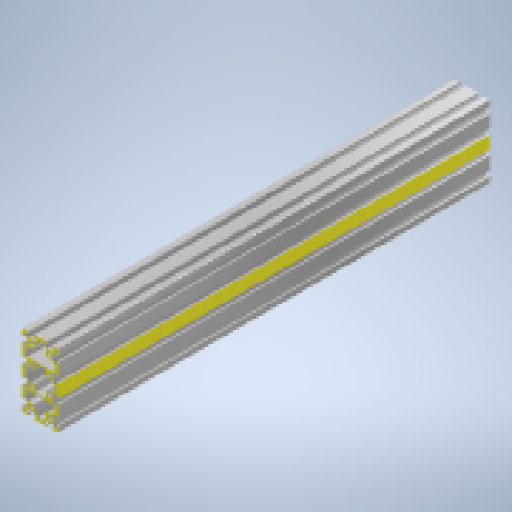
# Autodesk Inventor part: HFS5-4080-495
Saved by Autodesk Inventor 2024 (Build 280153000, 153)
## iProperties
Category: PARTsolutions
Company: MISUMI
Created: 2024-12-16
Part Number: HFS5-4080-495
Material: Aluminum 6061
Catalog Web Link: www.cadenas.de
Description: HFS5-2060, HFS5-2080, HFS5-4060, HFS5-4080, NFS5-2060, NFS5-2080, NFS5-4060, NFS5-4080-HFS5 Series Aluminum Extrusions 20mm Square -3 or more slots-
Vendor: MISUMI
Document SubType Name: Modeling
Designer: psAdmin
Manufacturer: MISUMI
Mass: 1327.09 g
Surface Area: 4398.43 cm^2
Volume: 491.514 cm^3
Density: 2.7 g/cm^3
Appearance: Aluminum - Flat
PSOL_IDENT_0: {$CADENAS_DATA/23d-libs/misumi/metric/38_al_extrusions_blackets/5/hfs5_2060.prj},622 {VTYP=3D},{NB=H
PSOL_IDENT_1: FS5-4080-495},{LINA=HFS5-4080-495},{NN=HFS5-2060, HFS5-2080, HFS5-4060, HFS5-4080, NFS5-2060, NFS5-2
PSOL_IDENT_2: 080, NFS5-4060, NFS5-4080},{DATE=08.05.2023 08:44:46},{GEOMDATE=27.07.2021 03:20:00},{VERSION=},{LIN
PSOL_IDENT_3: EID=220},{WBVAR=L,ALT1,ALT2,ALT4,ALT5,CP5,DL5,DR5,ALT6,ALT9,ALT10,ALT11,HP6,NHL6,DL6,NHR6,DR6,ALT7,A
PSOL_IDENT_4: LT8,NH9,AH,BH,CH,DH,EH,NH10,AV,BV,CV,DV,EV,NH11,AP,BP,CP,DP,EP,ALT12,ALT13,Z,NH12,XA,XB,XC,XD,XE,NH1
PSOL_IDENT_5: 3,YA,YB,YC,YD,YE,ALT16,HP16,DL16,DR16,ALT17,HQ17,JLP,ALT18,HQ18,KLP,ALT20},{WBNUMERIC=L,NH9,AH,BH,CH
PSOL_IDENT_6: ,DH,EH,NH10,AV,BV,CV,DV,EV,NH11,AP,BP,CP,DP,EP,NH12,XA,XB,XC,XD,XE,NH13,YA,YB,YC,YD,YE,HQ17,JLP,HQ18
PSOL_IDENT_7: ,KLP}  {NB=HFS5-4080-495},{LINA=HFS5-4080-495},{KT=DUMMY},{PN=HFS5-4080-495},{TPS=HFS5-4080},{MAT=A6
PSOL_IDENT_8: N01SS-T5 Aluminum Alloy},{ST=Clear Anodize},{FRMW=40},{FRMH=80},{FRD=4.2},{L=495},{MASS=2.69},{SA=99
PSOL_IDENT_9: 4},{LX=18.29x10^4},{LY=63.3x10^4},{ALT1=},{M1=0},{DPL1=0},{DPR1=0},{ALT1PN=},{ALT2=},{ALT2ALG= '','w
PSOL_IDENT_10: /o End Tapping (Heli-Coil Insert)','LHP','with LHP (Tapping on the Left (Heli-Coil Insert))','RHP','
PSOL_IDENT_11: with RHP (Tapping on the Right (Heli-Coil Insert))','HPW','with HPW (Tapping on Both Ends (Heli-Coil
PSOL_IDENT_12: Insert))' },{M2=0},{DP2=0},{ALT2PN=},{ALT4=},{ALT4ALG= '', 'w/o SC (High Precision Cut)', 'SC', 'wi
PSOL_IDENT_13: th SC (High Precision Cut)' },{ALT4PN=},{ALT5=},{ALT5ALG= '','w/o 45 Degree Cut','1','with 45 Degree
PSOL_IDENT_14: Cut' },{CP5=},{CP5ALG= '','N/A' },{DL5=},{DL5ALG= '','N/A' },{DR5=},{DR5ALG= '','N/A' },{FRMLALT5=0
PSOL_IDENT_15: },{FRMRALT5=0},{ALT5PN=},{ALT6=},{ALT6ALG= '','w/o Fastening Location Wrench Access Hole Alterations'
PSOL_IDENT_16: ,'1','with Fastening Location Wrench Access Hole Alterations' },{ALT9=},{ALT9ALG= '','w/o Location S
PSOL_IDENT_17: pecified Wrench Access Hole Alteratons (Horizontal)','1','with Location Specified Wrench Access Hole
PSOL_IDENT_18: Alteratons (Horizontal)' },{ALT10=},{ALT10ALG= '','w/o Location Specified Wrench Access Hole Altera
PSOL_IDENT_19: tons (Vertical)','1','with Location Specified Wrench Access Hole Alteratons (Vertical)' },{ALT11=},{
PSOL_IDENT_20: ALT11ALG= '','w/o Location Specified Wrench Access Hole Alteratons (Crisscross)','1','with Location
PSOL_IDENT_21: Specified Wrench Access Hole Alteratons (Crisscross)' },{DD6=0.00},{DD6ALG=0},{HP6=},{HP6ALG= '','N/
PSOL_IDENT_22: A' },{NHL6=},{NHL6ALG= '','N/A' },{DL6=},{DL6ALG= '','N/A' },{NHR6=},{NHR6ALG= '','N/A' },{DR6=},{DR
PSOL_IDENT_23: 6ALG= '','N/A' },{DD6PN=},{HL6=0},{HL6D=0},{HR6=0},{HR6D=0},{J6=0},{J6D=0},{K6=0},{K6D=0},{ALT7=},{A
PSOL_IDENT_24: LT7ALG= '','N/A' },{ALT8=},{ALT8ALG= '','N/A' },{ALT678PN=},{NH9=0},{NH9MAX=5},{NH9ALG=[0]},{AH=0.0}
PSOL_IDENT_25: ,{AHMIN=7},{AHMAX=490},{AHALG=[0]},{BH=0.0},{BHMIN=2},{BHMAX=492},{BHALG=[0]},{CH=0.0},{CHMIN=2},{CH
PSOL_IDENT_26: MAX=494},{CHALG=[0]},{DH=0.0},{DHMIN=2},{DHMAX=496},{DHALG=[0]},{EH=0.0},{EHMIN=2},{EHMAX=488},{EHAL
PSOL_IDENT_27: G=[0]},{NH10=0},{NH10MAX=5},{NH10ALG=[0]},{AV=0.0},{AVMIN=7},{AVMAX=490},{AVALG=[0]},{BV=0.0},{BVMIN=
PSOL_IDENT_28: 2},{BVMAX=492},{BVALG=[0]},{CV=0.0},{CVMIN=2},{CVMAX=494},{CVALG=[0]},{DV=0.0},{DVMIN=2},{DVMAX=496}
PSOL_IDENT_29: ,{DVALG=[0]},{EV=0.0},{EVMIN=2},{EVMAX=488},{EVALG=[0]},{NH11=0},{NH11MAX=5},{NH11ALG=[0]},{AP=0.0},
PSOL_IDENT_30: {APMIN=7},{APMAX=490},{APALG=[0]},{BP=0.0},{BPMIN=2},{BPMAX=492},{BPALG=[0]},{CP=0.0},{CPMIN=2},{CPM
PSOL_IDENT_31: AX=494},{CPALG=[0]},{DP=0.0},{DPMIN=2},{DPMAX=496},{DPALG=[0]},{EP=0.0},{EPMIN=2},{EPMAX=488},{EPALG=
PSOL_IDENT_32: [0]},{ALT9PN=},{ALT10PN=},{ALT11PN=},{ALT91011PN=},{ALT12=},{ALT12ALG= '','w/o Counterbore Hole in S
PSOL_IDENT_33: pecified Position (Vertical)','1','with Counterbore Hole in Specified Position (Vertical)' },{ALT13=
PSOL_IDENT_34: },{ALT13ALG= '','w/o Counterbore Hole in Specified Position (Horizontal)','1','with Counterbore Hole
PSOL_IDENT_35: in Specified Position (Horizontal)' },{Z=},{ZALG= '','N/A' },{DD12=0.0},{DD112=0.0},{NH12=0},{NH12M
PSOL_IDENT_36: AX=5},{NH12ALG=[0]},{XA=0.0},{XAMIN=7},{XAMAX=490},{XAALG=[0]},{XB=0.0},{XBMIN=2},{XBMAX=492},{XBALG=
PSOL_IDENT_37: [0]},{XC=0.0},{XCMIN=2},{XCMAX=494},{XCALG=[0]},{XD=0.0},{XDMIN=2},{XDMAX=496},{XDALG=[0]},{XE=0.0},
PSOL_IDENT_38: {XEMIN=2},{XEMAX=488},{XEALG=[0]},{NH13=0},{NH13MAX=5},{NH13ALG=[0]},{YA=0.0},{YAMIN=7},{YAMAX=490},
PSOL_IDENT_39: {YAALG=[0]},{YB=0.0},{YBMIN=2},{YBMAX=492},{YBALG=[0]},{YC=0.0},{YCMIN=2},{YCMAX=494},{YCALG=[0]},{Y
PSOL_IDENT_40: D=0.0},{YDMIN=2},{YDMAX=496},{YDALG=[0]},{YE=0.0},{YEMIN=2},{YEMAX=488},{YEALG=[0]},{ALT12PN=},{ALT1
PSOL_IDENT_41: 3PN=},{ALT1213PN=},{ALT16=},{ALT16ALG= '','w/o M Type Hole Alteration','1','with M Type Hole Alterat
PSOL_IDENT_42: ion' },{HP16=},{HP16ALG= '','N/A' },{DL16=},{DL16ALG= '','N/A' },{DR16=},{DR16ALG= '','N/A' },{H116=
PSOL_IDENT_43: 0},{D16=0.0},{ALT16PN=},{ALT17=},{ALT17ALG= '','w/o L Type Hole Alteration (Top)','1','with L Type H
PSOL_IDENT_44: ole Alteration (Top)' },{HQ17=0},{HQ17ALG=0},{JLP=0},{JLPMIN=4.9},{JLPMAX=0},{JLPALG=[0]},{L17=0},{D
PSOL_IDENT_45: 17=0.0},{ALT17PN=},{ALT18=},{ALT18ALG= '','w/o L Type Hole Alteration (Bottom)','1','with L Type Hol
PSOL_IDENT_46: e Alteration (Bottom)' },{HQ18=0},{HQ18ALG=0},{KLP=0},{KLPMIN=4.9},{KLPMAX=0},{KLPALG=[0]},{L18=0},{
PSOL_IDENT_47: D18=0.0},{ALT18PN=},{ALT20=},{ALT20PN=},{ERRORALT01=OK},{ERRORALT02=OK},{ERRORALT05=OK},{ERRORALT060
PSOL_IDENT_48: 91=OK},{ERRORALT06092=OK},{ERRORALT06093=OK},{ERRORALT06094=OK},{ERRORALT06101=OK},{ERRORALT06102=OK
PSOL_IDENT_49: },{ERRORALT06103=OK},{ERRORALT06104=OK},{ERRORALT06111=OK},{ERRORALT06112=OK},{ERRORALT06113=OK},{ER
PSOL_IDENT_50: RORALT06114=OK},{ERRORALT06121=OK},{ERRORALT06122=OK},{ERRORALT06123=OK},{ERRORALT06124=OK},{ERRORAL
PSOL_IDENT_51: T06131=OK},{ERRORALT06132=OK},{ERRORALT06133=OK},{ERRORALT06134=OK},{ERRORALT0616=OK},{ERRORALT06171=
PSOL_IDENT_52: OK},{ERRORALT06172=OK},{ERRORALT06173=OK},{ERRORALT06181=OK},{ERRORALT06182=OK},{ERRORALT06183=OK},{
PSOL_IDENT_53: ERRORALT0911=OK},{ERRORALT0913=OK},{ERRORALT0916=OK},{ERRORALT0917=OK},{ERRORALT0918=OK},{ERRORALT10
PSOL_IDENT_54: 11=OK},{ERRORALT1012=OK},{ERRORALT1016=OK},{ERRORALT1017=OK},{ERRORALT1018=OK},{ERRORALT1112=OK},{ER
PSOL_IDENT_55: RORALT1113=OK},{ERRORALT1116=OK},{ERRORALT1117=OK},{ERRORALT1118=OK},{ERRORALT1216=OK},{ERRORALT1217=
PSOL_IDENT_56: OK},{ERRORALT1218=OK},{ERRORALT1316=OK},{ERRORALT1317=OK},{ERRORALT1318=OK},{ERRORALT1617=OK},{ERROR
PSOL_IDENT_57: ALT1618=OK},{ERRORPN=},{TFW=0}
NB: HFS5-4080-495
NN: HFS5-2060, HFS5-2080, HFS5-4060, HFS5-4080, NFS5-2060, NFS5-2080, NFS5-4060, NFS5-4080
NT: HFS5 Series Aluminum Extrusions 20mm Square -3 or more slots-
NBSYN: $PN.
LINA: HFS5-4080-495
CATALOG: Misumi
PN: HFS5-4080-495
TPS: HFS5-4080
MAT: A6N01SS-T5 Aluminum Alloy
ST: Clear Anodize
L: 495
MASS: 2.69
SA: 994
LX: 18.29x10^4
LY: 63.3x10^4
ALT1: w/o End Tapping
M1: 0
DPL1: 0
DPR1: 0
ALT2: w/o End Tapping (Heli-Coil Insert)
M2: 0
DP2: 0
ALT4: w/o SC (High Precision Cut)
ALT5: w/o 45 Degree Cut
CP5: N/A
DL5: N/A
DR5: N/A
ALT6: w/o Fastening Location Wrench Access Hole Alterations
ALT9: w/o Location Specified Wrench Access Hole Alteratons (Horizontal)
ALT10: w/o Location Specified Wrench Access Hole Alteratons (Vertical)
ALT11: w/o Location Specified Wrench Access Hole Alteratons (Crisscross)
DD6: 0
HP6: N/A
NHL6: N/A
DL6: N/A
NHR6: N/A
DR6: N/A
HL6D: 0
HR6D: 0
J6D: 0
K6D: 0
ALT7: N/A
ALT8: N/A
NH9: 0
AH: 0
BH: 0
CH: 0
DH: 0
EH: 0
NH10: 0
AV: 0
BV: 0
CV: 0
DV: 0
EV: 0
NH11: 0
AP: 0
BP: 0
CP: 0
DP: 0
EP: 0
ALT12: w/o Counterbore Hole in Specified Position (Vertical)
ALT13: w/o Counterbore Hole in Specified Position (Horizontal)
Z: N/A
DD12: 0
DD112: 0
NH12: 0
XA: 0
XB: 0
XC: 0
XD: 0
XE: 0
NH13: 0
YA: 0
YB: 0
YC: 0
YD: 0
YE: 0
ALT16: w/o M Type Hole Alteration
HP16: N/A
DL16: N/A
DR16: N/A
H116: 0
D16: 0
ALT17: w/o L Type Hole Alteration (Top)
HQ17: 0
JLP: 0
D17: 0
ALT18: w/o L Type Hole Alteration (Bottom)
HQ18: 0
KLP: 0
D18: 0
ALT20: w/o CW (End Face C Chamfering)
SUPPLIER: MISUMI
ARTICLENO: HFS5-4080-495
BOMINFO: HFS5-4080-495
CREATOR: CADENAS GmbH
Title: HFS5-4080-495
Author: Cadenas PARTsolutions
Comments: HFS5 Series Aluminum Extrusions 20mm Square -3 or more slots-
Autodesk Inventor part; units mm, degrees
ref_plane "YZ Plane" through (0, 0, 0) normal (1, 0, 0) x (0, 1, 0)
ref_plane "XZ Plane" through (0, 0, 0) normal (0, 1, 0) x (-1, 0, 0)
ref_plane "XY Plane" through (0, 0, 0) normal (0, 0, 1) x (1, 0, 0)
sketch "Sketch_1" plane through (0, 0, 0) normal (0, 0, 1) x (1, 0, 0)
  line L0 (-20, -27) -> (-18, -27)
  line L1 (-18, -27) -> (-18, -24)
  line L2 (-18, -24) -> (-17.0607, -24)
  line L3 (-17.0607, -24) -> (-14, -27.0607)
  line L4 (-14, -27.0607) -> (-14, -29.4804)
  line L5 (-14, -29.4804) -> (-13.7, -30)
  line L6 (-13.7, -30) -> (-14, -30.5196)
  line L7 (-14, -30.5196) -> (-14, -32.9393)
  line L8 (-14, -32.9393) -> (-17.0607, -36)
  line L9 (-17.0607, -36) -> (-18, -36)
  line L10 (-18, -36) -> (-18, -33)
  line L11 (-18, -33) -> (-20, -33)
  line L12 (-20, -33) -> (-20, -39)
  arc A0 (-20, -39) -> (-19, -40) centre (-19, -39) ccw
  line L13 (-19, -40) -> (-13, -40)
  line L14 (-13, -40) -> (-13, -38)
  line L15 (-13, -38) -> (-16, -38)
  line L16 (-16, -38) -> (-16, -37.0607)
  line L17 (-16, -37.0607) -> (-12.9393, -34)
  line L18 (-12.9393, -34) -> (-10.5196, -34)
  line L19 (-10.5196, -34) -> (-10, -33.7)
  line L20 (-10, -33.7) -> (-9.4804, -34)
  line L21 (-9.4804, -34) -> (-7.0607, -34)
  line L22 (-7.0607, -34) -> (-4, -37.0607)
  line L23 (-4, -37.0607) -> (-4, -38)
  line L24 (-4, -38) -> (-7, -38)
  line L25 (-7, -38) -> (-7, -40)
  line L26 (-7, -40) -> (7, -40)
  line L27 (7, -40) -> (7, -38)
  line L28 (7, -38) -> (4, -38)
  line L29 (4, -38) -> (4, -37.0607)
  line L30 (4, -37.0607) -> (7.0607, -34)
  line L31 (7.0607, -34) -> (9.4804, -34)
  line L32 (9.4804, -34) -> (10, -33.7)
  line L33 (10, -33.7) -> (10.5196, -34)
  line L34 (10.5196, -34) -> (12.9393, -34)
  line L35 (12.9393, -34) -> (16, -37.0607)
  line L36 (16, -37.0607) -> (16, -38)
  line L37 (16, -38) -> (13, -38)
  line L38 (13, -38) -> (13, -40)
  line L39 (13, -40) -> (19, -40)
  arc A1 (19, -40) -> (20, -39) centre (19, -39) ccw
  line L40 (20, -39) -> (20, -33)
  line L41 (20, -33) -> (18, -33)
  line L42 (18, -33) -> (18, -36)
  line L43 (18, -36) -> (17.0607, -36)
  line L44 (17.0607, -36) -> (14, -32.9393)
  line L45 (14, -32.9393) -> (14, -30.5196)
  line L46 (14, -30.5196) -> (13.7, -30)
  line L47 (13.7, -30) -> (14, -29.4804)
  line L48 (14, -29.4804) -> (14, -27.0607)
  line L49 (14, -27.0607) -> (17.0607, -24)
  line L50 (17.0607, -24) -> (18, -24)
  line L51 (18, -24) -> (18, -27)
  line L52 (18, -27) -> (20, -27)
  line L53 (20, -27) -> (20, -13)
  line L54 (20, -13) -> (18, -13)
  line L55 (18, -13) -> (18, -16)
  line L56 (18, -16) -> (17.0607, -16)
  line L57 (17.0607, -16) -> (14, -12.9393)
  line L58 (14, -12.9393) -> (14, -10.5196)
  line L59 (14, -10.5196) -> (13.7, -10)
  line L60 (13.7, -10) -> (14, -9.4804)
  line L61 (14, -9.4804) -> (14, -7.0607)
  line L62 (14, -7.0607) -> (17.0607, -4)
  line L63 (17.0607, -4) -> (18, -4)
  line L64 (18, -4) -> (18, -7)
  line L65 (18, -7) -> (20, -7)
  line L66 (20, -7) -> (20, 7)
  line L67 (20, 7) -> (18, 7)
  line L68 (18, 7) -> (18, 4)
  line L69 (18, 4) -> (17.0607, 4)
  line L70 (17.0607, 4) -> (14, 7.0607)
  line L71 (14, 7.0607) -> (14, 9.4804)
  line L72 (14, 9.4804) -> (13.7, 10)
  line L73 (13.7, 10) -> (14, 10.5196)
  line L74 (14, 10.5196) -> (14, 12.9393)
  line L75 (14, 12.9393) -> (17.0607, 16)
  line L76 (17.0607, 16) -> (18, 16)
  line L77 (18, 16) -> (18, 13)
  line L78 (18, 13) -> (20, 13)
  line L79 (20, 13) -> (20, 27)
  line L80 (20, 27) -> (18, 27)
  line L81 (18, 27) -> (18, 24)
  line L82 (18, 24) -> (17.0607, 24)
  line L83 (17.0607, 24) -> (14, 27.0607)
  line L84 (14, 27.0607) -> (14, 29.4804)
  line L85 (14, 29.4804) -> (13.7, 30)
  line L86 (13.7, 30) -> (14, 30.5196)
  line L87 (14, 30.5196) -> (14, 32.9393)
  line L88 (14, 32.9393) -> (17.0607, 36)
  line L89 (17.0607, 36) -> (18, 36)
  line L90 (18, 36) -> (18, 33)
  line L91 (18, 33) -> (20, 33)
  line L92 (20, 33) -> (20, 39)
  arc A2 (20, 39) -> (19, 40) centre (19, 39) ccw
  line L93 (19, 40) -> (13, 40)
  line L94 (13, 40) -> (13, 38)
  line L95 (13, 38) -> (16, 38)
  line L96 (16, 38) -> (16, 37.0607)
  line L97 (16, 37.0607) -> (12.9393, 34)
  line L98 (12.9393, 34) -> (10.5196, 34)
  line L99 (10.5196, 34) -> (10, 33.7)
  line L100 (10, 33.7) -> (9.4804, 34)
  line L101 (9.4804, 34) -> (7.0607, 34)
  line L102 (7.0607, 34) -> (4, 37.0607)
  line L103 (4, 37.0607) -> (4, 38)
  line L104 (4, 38) -> (7, 38)
  line L105 (7, 38) -> (7, 40)
  line L106 (7, 40) -> (-7, 40)
  line L107 (-7, 40) -> (-7, 38)
  line L108 (-7, 38) -> (-4, 38)
  line L109 (-4, 38) -> (-4, 37.0607)
  line L110 (-4, 37.0607) -> (-7.0607, 34)
  line L111 (-7.0607, 34) -> (-9.4804, 34)
  line L112 (-9.4804, 34) -> (-10, 33.7)
  line L113 (-10, 33.7) -> (-10.5196, 34)
  line L114 (-10.5196, 34) -> (-12.9393, 34)
  line L115 (-12.9393, 34) -> (-16, 37.0607)
  line L116 (-16, 37.0607) -> (-16, 38)
  line L117 (-16, 38) -> (-13, 38)
  line L118 (-13, 38) -> (-13, 40)
  line L119 (-13, 40) -> (-19, 40)
  arc A3 (-19, 40) -> (-20, 39) centre (-19, 39) ccw
  line L120 (-20, 39) -> (-20, 33)
  line L121 (-20, 33) -> (-18, 33)
  line L122 (-18, 33) -> (-18, 36)
  line L123 (-18, 36) -> (-17.0607, 36)
  line L124 (-17.0607, 36) -> (-14, 32.9393)
  line L125 (-14, 32.9393) -> (-14, 30.5196)
  line L126 (-14, 30.5196) -> (-13.7, 30)
  line L127 (-13.7, 30) -> (-14, 29.4804)
  line L128 (-14, 29.4804) -> (-14, 27.0607)
  line L129 (-14, 27.0607) -> (-17.0607, 24)
  line L130 (-17.0607, 24) -> (-18, 24)
  line L131 (-18, 24) -> (-18, 27)
  line L132 (-18, 27) -> (-20, 27)
  line L133 (-20, 27) -> (-20, 13)
  line L134 (-20, 13) -> (-18, 13)
  line L135 (-18, 13) -> (-18, 16)
  line L136 (-18, 16) -> (-17.0607, 16)
  line L137 (-17.0607, 16) -> (-14, 12.9393)
  line L138 (-14, 12.9393) -> (-14, 10.5196)
  line L139 (-14, 10.5196) -> (-13.7, 10)
  line L140 (-13.7, 10) -> (-14, 9.4804)
  line L141 (-14, 9.4804) -> (-14, 7.0607)
  line L142 (-14, 7.0607) -> (-17.0607, 4)
  line L143 (-17.0607, 4) -> (-18, 4)
  line L144 (-18, 4) -> (-18, 7)
  line L145 (-18, 7) -> (-20, 7)
  line L146 (-20, 7) -> (-20, -7)
  line L147 (-20, -7) -> (-18, -7)
  line L148 (-18, -7) -> (-18, -4)
  line L149 (-18, -4) -> (-17.0607, -4)
  line L150 (-17.0607, -4) -> (-14, -7.0607)
  line L151 (-14, -7.0607) -> (-14, -9.4804)
  line L152 (-14, -9.4804) -> (-13.7, -10)
  line L153 (-13.7, -10) -> (-14, -10.5196)
  line L154 (-14, -10.5196) -> (-14, -12.9393)
  line L155 (-14, -12.9393) -> (-17.0607, -16)
  line L156 (-17.0607, -16) -> (-18, -16)
  line L157 (-18, -16) -> (-18, -13)
  line L158 (-18, -13) -> (-20, -13)
  line L159 (-20, -13) -> (-20, -27)
  line L160 (-16.5, 17.5607) -> (-14.4393, 15.5)
  line L161 (-14.4393, 15.5) -> (14.4393, 15.5)
  line L162 (14.4393, 15.5) -> (16.5, 17.5607)
  line L163 (16.5, 17.5607) -> (16.5, 22.4393)
  line L164 (16.5, 22.4393) -> (12.9393, 26)
  line L165 (12.9393, 26) -> (9, 26)
  arc A4 (6, 29) -> (9, 26) centre (9, 29) ccw
  line L166 (6, 29) -> (6, 32.9393)
  line L167 (6, 32.9393) -> (2.4393, 36.5)
  line L168 (2.4393, 36.5) -> (-2.4393, 36.5)
  line L169 (-2.4393, 36.5) -> (-6, 32.9393)
  line L170 (-6, 32.9393) -> (-6, 29)
  arc A5 (-9, 26) -> (-6, 29) centre (-9, 29) ccw
  line L171 (-9, 26) -> (-12.9393, 26)
  line L172 (-12.9393, 26) -> (-16.5, 22.4393)
  line L173 (-16.5, 22.4393) -> (-16.5, 17.5607)
  line L174 (-16.5, -2.4393) -> (-11.2996, -7.6397)
  arc A6 (-11.3353, -8.3792) -> (-11.2996, -7.6397) centre (-11.6532, -7.9933) ccw
  arc A7 (-11.3353, -8.3792) -> (-8.6199, -8.4172) centre (-10, -10) ccw
  arc A8 (-8.7243, -7.7904) -> (-8.6199, -8.4172) centre (-8.2913, -8.0404) ccw
  line L175 (-8.7243, -7.7904) -> (-7.6906, -6)
  line L176 (-7.6906, -6) -> (-6, -6)
  line L177 (-6, -6) -> (-6, -14)
  line L178 (-6, -14) -> (6, -14)
  line L179 (6, -14) -> (6, -6)
  line L180 (6, -6) -> (7.6906, -6)
  line L181 (7.6906, -6) -> (8.7243, -7.7904)
  arc A9 (8.6199, -8.4172) -> (8.7243, -7.7904) centre (8.2913, -8.0404) ccw
  arc A10 (8.6199, -8.4172) -> (11.3353, -8.3792) centre (10, -10) ccw
  arc A11 (11.2996, -7.6397) -> (11.3353, -8.3792) centre (11.6532, -7.9933) ccw
  line L182 (11.2996, -7.6397) -> (16.5, -2.4393)
  line L183 (16.5, -2.4393) -> (16.5, 2.4393)
  line L184 (16.5, 2.4393) -> (11.2996, 7.6397)
  arc A12 (11.3353, 8.3792) -> (11.2996, 7.6397) centre (11.6532, 7.9933) ccw
  arc A13 (11.3353, 8.3792) -> (8.6199, 8.4172) centre (10, 10) ccw
  arc A14 (8.7243, 7.7904) -> (8.6199, 8.4172) centre (8.2913, 8.0404) ccw
  line L185 (8.7243, 7.7904) -> (7.6906, 6)
  line L186 (7.6906, 6) -> (6, 6)
  line L187 (6, 6) -> (6, 14)
  line L188 (6, 14) -> (-6, 14)
  line L189 (-6, 14) -> (-6, 6)
  line L190 (-6, 6) -> (-7.6906, 6)
  line L191 (-7.6906, 6) -> (-8.7243, 7.7904)
  arc A15 (-8.6199, 8.4172) -> (-8.7243, 7.7904) centre (-8.2913, 8.0404) ccw
  arc A16 (-8.6199, 8.4172) -> (-11.3353, 8.3792) centre (-10, 10) ccw
  arc A17 (-11.2996, 7.6397) -> (-11.3353, 8.3792) centre (-11.6532, 7.9933) ccw
  line L192 (-11.2996, 7.6397) -> (-16.5, 2.4393)
  line L193 (-16.5, 2.4393) -> (-16.5, -2.4393)
  line L194 (-16.5, -17.5607) -> (-16.5, -22.4393)
  line L195 (-16.5, -22.4393) -> (-12.9393, -26)
  line L196 (-12.9393, -26) -> (-9, -26)
  arc A18 (-6, -29) -> (-9, -26) centre (-9, -29) ccw
  line L197 (-6, -29) -> (-6, -32.9393)
  line L198 (-6, -32.9393) -> (-2.4393, -36.5)
  line L199 (-2.4393, -36.5) -> (2.4393, -36.5)
  line L200 (2.4393, -36.5) -> (6, -32.9393)
  line L201 (6, -32.9393) -> (6, -29)
  arc A19 (9, -26) -> (6, -29) centre (9, -29) ccw
  line L202 (9, -26) -> (12.9393, -26)
  line L203 (12.9393, -26) -> (16.5, -22.4393)
  line L204 (16.5, -22.4393) -> (16.5, -17.5607)
  line L205 (16.5, -17.5607) -> (14.4393, -15.5)
  line L206 (14.4393, -15.5) -> (-14.4393, -15.5)
  line L207 (-14.4393, -15.5) -> (-16.5, -17.5607)
  constraints: 416 end point, 40 point on circle, 20 centre point
extrude "Extrusion1" add sketch "Sketch_1" against normal blind 475
sketch "Sketch2" plane through (0, 0, 0) normal (0, 0, 1) x (1, 0, 0)
  point P0 (10, 30)
hole "Hole1" at (10, 30, 0) direction (0, 0, -1) diameter 4.2 depth 495
pattern_linear "Rectangular Pattern1" count 2 spacing 20 along (-1, 0, 0) count 2 spacing 60 along (0, -1, 0) of "Hole1"
body "Solid1"
